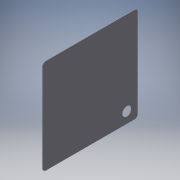
# Autodesk Inventor part: NewFront_C
Saved by Autodesk Inventor 2017 (Build 210142000, 142)
## iProperties
Created: 2019-07-06
Part Number: NewFront_C
Material: Generic
Document SubType Name: Modeling
Designer: DDeGo
Density: 1 g/cm^3
Appearance: Default
Author: DDeGo
Autodesk Inventor part; units mm, degrees
ref_plane "YZ Plane" through (0, 0, 0) normal (1, 0, 0) x (0, 1, 0)
ref_plane "XZ Plane" through (0, 0, 0) normal (0, 1, 0) x (-1, 0, 0)
ref_plane "XY Plane" through (0, 0, 0) normal (0, 0, 1) x (1, 0, 0)
sketch "Sketch1" plane through (0, 0, 0) normal (1, 0, 0) x (0, 1, 0)
  line L0 (0, 13.5) -> (156.5, 13.5) construction
  line L1 (170, 0) -> (170, -156.5) construction
  line L2 (156.5, -170) -> (0, -170) construction
  line L3 (-13.5, -156.5) -> (-13.5, 0) construction
  arc A0 (170, 0) -> (156.5, 13.5) centre (156.5, 0) ccw construction
  arc A1 (156.5, -170) -> (170, -156.5) centre (156.5, -156.5) ccw construction
  arc A2 (-13.5, -156.5) -> (0, -170) centre (0, -156.5) ccw construction
  arc A3 (0, 13.5) -> (-13.5, 0) centre (0, 0) ccw construction
  line L4 (26.5, -21.5) -> (130, -21.5)
  line L5 (135, -26.5) -> (135, -130)
  line L6 (130, -135) -> (26.5, -135)
  line L7 (21.5, -130) -> (21.5, -26.5)
  arc A4 (26.5, -21.5) -> (21.5, -26.5) centre (26.5, -26.5) ccw
  arc A5 (21.5, -130) -> (26.5, -135) centre (26.5, -130) ccw
  arc A6 (130, -135) -> (135, -130) centre (130, -130) ccw
  arc A7 (135, -26.5) -> (130, -21.5) centre (130, -26.5) ccw
  line L8 (156.5, 5.5) -> (0, 5.5)
  arc A8 (0, 5.5) -> (-5.5, 0) centre (0, 0) ccw
  line L9 (-5.5, 0) -> (-5.5, -156.5)
  arc A9 (-5.5, -156.5) -> (0, -162) centre (0, -156.5) ccw
  line L10 (0, -162) -> (156.5, -162)
  arc A10 (156.5, -162) -> (162, -156.5) centre (156.5, -156.5) ccw
  line L11 (162, -156.5) -> (162, 0)
  arc A11 (162, 0) -> (156.5, 5.5) centre (156.5, 0) ccw
  line L12 (17.5, 5.5) -> (17.5, -10.5) construction
  line L13 (14.5, 5.5) -> (14.5, -10.5)
  line L14 (20.5, -10.5) -> (20.5, 5.5)
  arc A12 (20.5, 5.5) -> (14.5, 5.5) centre (17.5, 5.5) ccw
  arc A13 (14.5, -10.5) -> (20.5, -10.5) centre (17.5, -10.5) ccw
  line L15 (31.5455, -10.5) -> (31.5455, 5.5)
  line L16 (28.5455, 5.5) -> (28.5455, -10.5) construction
  arc A14 (25.5455, -10.5) -> (31.5455, -10.5) centre (28.5455, -10.5) ccw
  arc A15 (31.5455, 5.5) -> (25.5455, 5.5) centre (28.5455, 5.5) ccw
  line L17 (25.5455, 5.5) -> (25.5455, -10.5)
  line L18 (42.5909, -10.5) -> (42.5909, 5.5)
  line L19 (39.5909, 5.5) -> (39.5909, -10.5) construction
  arc A16 (36.5909, -10.5) -> (42.5909, -10.5) centre (39.5909, -10.5) ccw
  arc A17 (42.5909, 5.5) -> (36.5909, 5.5) centre (39.5909, 5.5) ccw
  line L20 (36.5909, 5.5) -> (36.5909, -10.5)
  line L21 (53.6364, -10.5) -> (53.6364, 5.5)
  line L22 (50.6364, 5.5) -> (50.6364, -10.5) construction
  arc A18 (47.6364, -10.5) -> (53.6364, -10.5) centre (50.6364, -10.5) ccw
  arc A19 (53.6364, 5.5) -> (47.6364, 5.5) centre (50.6364, 5.5) ccw
  line L23 (47.6364, 5.5) -> (47.6364, -10.5)
  line L24 (64.6818, -10.5) -> (64.6818, 5.5)
  line L25 (61.6818, 5.5) -> (61.6818, -10.5) construction
  arc A20 (58.6818, -10.5) -> (64.6818, -10.5) centre (61.6818, -10.5) ccw
  arc A21 (64.6818, 5.5) -> (58.6818, 5.5) centre (61.6818, 5.5) ccw
  line L26 (58.6818, 5.5) -> (58.6818, -10.5)
  line L27 (75.7273, -10.5) -> (75.7273, 5.5)
  line L28 (72.7273, 5.5) -> (72.7273, -10.5) construction
  arc A22 (69.7273, -10.5) -> (75.7273, -10.5) centre (72.7273, -10.5) ccw
  arc A23 (75.7273, 5.5) -> (69.7273, 5.5) centre (72.7273, 5.5) ccw
  line L29 (69.7273, 5.5) -> (69.7273, -10.5)
  line L30 (86.7727, -10.5) -> (86.7727, 5.5)
  line L31 (83.7727, 5.5) -> (83.7727, -10.5) construction
  arc A24 (80.7727, -10.5) -> (86.7727, -10.5) centre (83.7727, -10.5) ccw
  arc A25 (86.7727, 5.5) -> (80.7727, 5.5) centre (83.7727, 5.5) ccw
  line L32 (80.7727, 5.5) -> (80.7727, -10.5)
  line L33 (97.8182, -10.5) -> (97.8182, 5.5)
  line L34 (94.8182, 5.5) -> (94.8182, -10.5) construction
  arc A26 (91.8182, -10.5) -> (97.8182, -10.5) centre (94.8182, -10.5) ccw
  arc A27 (97.8182, 5.5) -> (91.8182, 5.5) centre (94.8182, 5.5) ccw
  line L35 (91.8182, 5.5) -> (91.8182, -10.5)
  line L36 (108.8636, -10.5) -> (108.8636, 5.5)
  line L37 (105.8636, 5.5) -> (105.8636, -10.5) construction
  arc A28 (102.8636, -10.5) -> (108.8636, -10.5) centre (105.8636, -10.5) ccw
  arc A29 (108.8636, 5.5) -> (102.8636, 5.5) centre (105.8636, 5.5) ccw
  line L38 (102.8636, 5.5) -> (102.8636, -10.5)
  line L39 (119.9091, -10.5) -> (119.9091, 5.5)
  line L40 (116.9091, 5.5) -> (116.9091, -10.5) construction
  arc A30 (113.9091, -10.5) -> (119.9091, -10.5) centre (116.9091, -10.5) ccw
  arc A31 (119.9091, 5.5) -> (113.9091, 5.5) centre (116.9091, 5.5) ccw
  line L41 (113.9091, 5.5) -> (113.9091, -10.5)
  line L42 (130.9545, -10.5) -> (130.9545, 5.5)
  line L43 (127.9545, 5.5) -> (127.9545, -10.5) construction
  arc A32 (124.9545, -10.5) -> (130.9545, -10.5) centre (127.9545, -10.5) ccw
  arc A33 (130.9545, 5.5) -> (124.9545, 5.5) centre (127.9545, 5.5) ccw
  line L44 (124.9545, 5.5) -> (124.9545, -10.5)
  line L45 (142, -10.5) -> (142, 5.5)
  line L46 (139, 5.5) -> (139, -10.5) construction
  arc A34 (136, -10.5) -> (142, -10.5) centre (139, -10.5) ccw
  arc A35 (142, 5.5) -> (136, 5.5) centre (139, 5.5) ccw
  line L47 (136, 5.5) -> (136, -10.5)
  line L48 (26.5, -26.5) -> (130, -130) construction
  arc A36 (10.5, -86.7727) -> (10.5, -80.7727) centre (10.5, -83.7727) ccw
  arc A37 (10.5, -97.8182) -> (10.5, -91.8182) centre (10.5, -94.8182) ccw
  arc A38 (10.5, -119.9091) -> (10.5, -113.9091) centre (10.5, -116.9091) ccw
  arc A39 (10.5, -75.7273) -> (10.5, -69.7273) centre (10.5, -72.7273) ccw
  arc A40 (10.5, -64.6818) -> (10.5, -58.6818) centre (10.5, -61.6818) ccw
  arc A41 (10.5, -53.6364) -> (10.5, -47.6364) centre (10.5, -50.6364) ccw
  arc A42 (10.5, -42.5909) -> (10.5, -36.5909) centre (10.5, -39.5909) ccw
  arc A43 (10.5, -108.8636) -> (10.5, -102.8636) centre (10.5, -105.8636) ccw
  line L49 (10.5, -124.9545) -> (-5.5, -124.9545)
  line L50 (-5.5, -127.9545) -> (10.5, -127.9545) construction
  line L51 (-5.5, -130.9545) -> (10.5, -130.9545)
  arc A44 (-5.5, -124.9545) -> (-5.5, -130.9545) centre (-5.5, -127.9545) ccw
  line L52 (10.5, -136) -> (-5.5, -136)
  line L53 (-5.5, -139) -> (10.5, -139) construction
  arc A45 (-5.5, -136) -> (-5.5, -142) centre (-5.5, -139) ccw
  line L54 (-5.5, -142) -> (10.5, -142)
  arc A46 (10.5, -142) -> (10.5, -136) centre (10.5, -139) ccw
  arc A47 (10.5, -130.9545) -> (10.5, -124.9545) centre (10.5, -127.9545) ccw
  line L55 (-5.5, -119.9091) -> (10.5, -119.9091)
  line L56 (-5.5, -116.9091) -> (10.5, -116.9091) construction
  arc A48 (-5.5, -113.9091) -> (-5.5, -119.9091) centre (-5.5, -116.9091) ccw
  line L57 (10.5, -113.9091) -> (-5.5, -113.9091)
  line L58 (-5.5, -108.8636) -> (10.5, -108.8636)
  line L59 (-5.5, -105.8636) -> (10.5, -105.8636) construction
  line L60 (10.5, -102.8636) -> (-5.5, -102.8636)
  arc A49 (-5.5, -102.8636) -> (-5.5, -108.8636) centre (-5.5, -105.8636) ccw
  line L61 (-5.5, -86.7727) -> (10.5, -86.7727)
  line L62 (-5.5, -83.7727) -> (10.5, -83.7727) construction
  line L63 (10.5, -80.7727) -> (-5.5, -80.7727)
  arc A50 (-5.5, -80.7727) -> (-5.5, -86.7727) centre (-5.5, -83.7727) ccw
  line L64 (-5.5, -75.7273) -> (10.5, -75.7273)
  line L65 (-5.5, -72.7273) -> (10.5, -72.7273) construction
  line L66 (10.5, -69.7273) -> (-5.5, -69.7273)
  arc A51 (-5.5, -69.7273) -> (-5.5, -75.7273) centre (-5.5, -72.7273) ccw
  line L67 (-5.5, -64.6818) -> (10.5, -64.6818)
  line L68 (-5.5, -61.6818) -> (10.5, -61.6818) construction
  line L69 (10.5, -58.6818) -> (-5.5, -58.6818)
  arc A52 (-5.5, -58.6818) -> (-5.5, -64.6818) centre (-5.5, -61.6818) ccw
  line L70 (-5.5, -97.8182) -> (10.5, -97.8182)
  line L71 (-5.5, -94.8182) -> (10.5, -94.8182) construction
  line L72 (10.5, -91.8182) -> (-5.5, -91.8182)
  arc A53 (-5.5, -91.8182) -> (-5.5, -97.8182) centre (-5.5, -94.8182) ccw
  arc A54 (-5.5, -14.5) -> (-5.5, -20.5) centre (-5.5, -17.5) ccw
  line L73 (10.5, -14.5) -> (-5.5, -14.5)
  line L74 (-5.5, -17.5) -> (10.5, -17.5) construction
  line L75 (-5.5, -20.5) -> (10.5, -20.5)
  arc A55 (10.5, -20.5) -> (10.5, -14.5) centre (10.5, -17.5) ccw
  line L76 (-5.5, -28.5455) -> (10.5, -28.5455) construction
  line L77 (-5.5, -31.5455) -> (10.5, -31.5455)
  arc A56 (10.5, -31.5455) -> (10.5, -25.5455) centre (10.5, -28.5455) ccw
  arc A57 (-5.5, -36.5909) -> (-5.5, -42.5909) centre (-5.5, -39.5909) ccw
  line L78 (10.5, -36.5909) -> (-5.5, -36.5909)
  line L79 (-5.5, -39.5909) -> (10.5, -39.5909) construction
  arc A58 (-5.5, -25.5455) -> (-5.5, -31.5455) centre (-5.5, -28.5455) ccw
  line L80 (-5.5, -53.6364) -> (10.5, -53.6364)
  line L81 (-5.5, -50.6364) -> (10.5, -50.6364) construction
  arc A59 (-5.5, -47.6364) -> (-5.5, -53.6364) centre (-5.5, -50.6364) ccw
  line L82 (10.5, -47.6364) -> (-5.5, -47.6364)
  line L83 (-5.5, -42.5909) -> (10.5, -42.5909)
  line L84 (10.5, -25.5455) -> (-5.5, -25.5455)
  arc A60 (86.7727, -146) -> (80.7727, -146) centre (83.7727, -146) ccw
  arc A61 (97.8182, -146) -> (91.8182, -146) centre (94.8182, -146) ccw
  arc A62 (119.9091, -146) -> (113.9091, -146) centre (116.9091, -146) ccw
  arc A63 (75.7273, -146) -> (69.7273, -146) centre (72.7273, -146) ccw
  arc A64 (64.6818, -146) -> (58.6818, -146) centre (61.6818, -146) ccw
  arc A65 (53.6364, -146) -> (47.6364, -146) centre (50.6364, -146) ccw
  arc A66 (42.5909, -146) -> (36.5909, -146) centre (39.5909, -146) ccw
  arc A67 (108.8636, -146) -> (102.8636, -146) centre (105.8636, -146) ccw
  line L85 (124.9545, -146) -> (124.9545, -162)
  line L86 (127.9545, -162) -> (127.9545, -146) construction
  line L87 (130.9545, -162) -> (130.9545, -146)
  arc A68 (124.9545, -162) -> (130.9545, -162) centre (127.9545, -162) ccw
  line L88 (136, -146) -> (136, -162)
  line L89 (139, -162) -> (139, -146) construction
  arc A69 (136, -162) -> (142, -162) centre (139, -162) ccw
  line L90 (142, -162) -> (142, -146)
  arc A70 (142, -146) -> (136, -146) centre (139, -146) ccw
  arc A71 (130.9545, -146) -> (124.9545, -146) centre (127.9545, -146) ccw
  line L91 (119.9091, -162) -> (119.9091, -146)
  line L92 (116.9091, -162) -> (116.9091, -146) construction
  arc A72 (113.9091, -162) -> (119.9091, -162) centre (116.9091, -162) ccw
  line L93 (113.9091, -146) -> (113.9091, -162)
  line L94 (108.8636, -162) -> (108.8636, -146)
  line L95 (105.8636, -162) -> (105.8636, -146) construction
  line L96 (102.8636, -146) -> (102.8636, -162)
  arc A73 (102.8636, -162) -> (108.8636, -162) centre (105.8636, -162) ccw
  line L97 (86.7727, -162) -> (86.7727, -146)
  line L98 (83.7727, -162) -> (83.7727, -146) construction
  line L99 (80.7727, -146) -> (80.7727, -162)
  arc A74 (80.7727, -162) -> (86.7727, -162) centre (83.7727, -162) ccw
  line L100 (75.7273, -162) -> (75.7273, -146)
  line L101 (72.7273, -162) -> (72.7273, -146) construction
  line L102 (69.7273, -146) -> (69.7273, -162)
  arc A75 (69.7273, -162) -> (75.7273, -162) centre (72.7273, -162) ccw
  line L103 (64.6818, -162) -> (64.6818, -146)
  line L104 (61.6818, -162) -> (61.6818, -146) construction
  line L105 (58.6818, -146) -> (58.6818, -162)
  arc A76 (58.6818, -162) -> (64.6818, -162) centre (61.6818, -162) ccw
  line L106 (97.8182, -162) -> (97.8182, -146)
  line L107 (94.8182, -162) -> (94.8182, -146) construction
  line L108 (91.8182, -146) -> (91.8182, -162)
  arc A77 (91.8182, -162) -> (97.8182, -162) centre (94.8182, -162) ccw
  arc A78 (14.5, -162) -> (20.5, -162) centre (17.5, -162) ccw
  line L109 (14.5, -146) -> (14.5, -162)
  line L110 (17.5, -162) -> (17.5, -146) construction
  line L111 (20.5, -162) -> (20.5, -146)
  arc A79 (20.5, -146) -> (14.5, -146) centre (17.5, -146) ccw
  line L112 (28.5455, -162) -> (28.5455, -146) construction
  line L113 (31.5455, -162) -> (31.5455, -146)
  arc A80 (31.5455, -146) -> (25.5455, -146) centre (28.5455, -146) ccw
  arc A81 (36.5909, -162) -> (42.5909, -162) centre (39.5909, -162) ccw
  line L114 (36.5909, -146) -> (36.5909, -162)
  line L115 (39.5909, -162) -> (39.5909, -146) construction
  arc A82 (25.5455, -162) -> (31.5455, -162) centre (28.5455, -162) ccw
  line L116 (53.6364, -162) -> (53.6364, -146)
  line L117 (50.6364, -162) -> (50.6364, -146) construction
  arc A83 (47.6364, -162) -> (53.6364, -162) centre (50.6364, -162) ccw
  line L118 (47.6364, -146) -> (47.6364, -162)
  line L119 (42.5909, -162) -> (42.5909, -146)
  line L120 (25.5455, -146) -> (25.5455, -162)
  arc A84 (146, -69.7273) -> (146, -75.7273) centre (146, -72.7273) ccw
  arc A85 (146, -58.6818) -> (146, -64.6818) centre (146, -61.6818) ccw
  arc A86 (146, -36.5909) -> (146, -42.5909) centre (146, -39.5909) ccw
  arc A87 (146, -80.7727) -> (146, -86.7727) centre (146, -83.7727) ccw
  arc A88 (146, -91.8182) -> (146, -97.8182) centre (146, -94.8182) ccw
  arc A89 (146, -102.8636) -> (146, -108.8636) centre (146, -105.8636) ccw
  arc A90 (146, -113.9091) -> (146, -119.9091) centre (146, -116.9091) ccw
  arc A91 (146, -47.6364) -> (146, -53.6364) centre (146, -50.6364) ccw
  line L121 (146, -31.5455) -> (162, -31.5455)
  line L122 (162, -28.5455) -> (146, -28.5455) construction
  line L123 (162, -25.5455) -> (146, -25.5455)
  arc A92 (162, -31.5455) -> (162, -25.5455) centre (162, -28.5455) ccw
  line L124 (146, -20.5) -> (162, -20.5)
  line L125 (162, -17.5) -> (146, -17.5) construction
  arc A93 (162, -20.5) -> (162, -14.5) centre (162, -17.5) ccw
  line L126 (162, -14.5) -> (146, -14.5)
  arc A94 (146, -14.5) -> (146, -20.5) centre (146, -17.5) ccw
  arc A95 (146, -25.5455) -> (146, -31.5455) centre (146, -28.5455) ccw
  line L127 (162, -36.5909) -> (146, -36.5909)
  line L128 (162, -39.5909) -> (146, -39.5909) construction
  arc A96 (162, -42.5909) -> (162, -36.5909) centre (162, -39.5909) ccw
  line L129 (146, -42.5909) -> (162, -42.5909)
  line L130 (162, -47.6364) -> (146, -47.6364)
  line L131 (162, -50.6364) -> (146, -50.6364) construction
  line L132 (146, -53.6364) -> (162, -53.6364)
  arc A97 (162, -53.6364) -> (162, -47.6364) centre (162, -50.6364) ccw
  line L133 (162, -69.7273) -> (146, -69.7273)
  line L134 (162, -72.7273) -> (146, -72.7273) construction
  line L135 (146, -75.7273) -> (162, -75.7273)
  arc A98 (162, -75.7273) -> (162, -69.7273) centre (162, -72.7273) ccw
  line L136 (162, -80.7727) -> (146, -80.7727)
  line L137 (162, -83.7727) -> (146, -83.7727) construction
  line L138 (146, -86.7727) -> (162, -86.7727)
  arc A99 (162, -86.7727) -> (162, -80.7727) centre (162, -83.7727) ccw
  line L139 (162, -91.8182) -> (146, -91.8182)
  line L140 (162, -94.8182) -> (146, -94.8182) construction
  line L141 (146, -97.8182) -> (162, -97.8182)
  arc A100 (162, -97.8182) -> (162, -91.8182) centre (162, -94.8182) ccw
  line L142 (162, -58.6818) -> (146, -58.6818)
  line L143 (162, -61.6818) -> (146, -61.6818) construction
  line L144 (146, -64.6818) -> (162, -64.6818)
  arc A101 (162, -64.6818) -> (162, -58.6818) centre (162, -61.6818) ccw
  arc A102 (162, -142) -> (162, -136) centre (162, -139) ccw
  line L145 (146, -142) -> (162, -142)
  line L146 (162, -139) -> (146, -139) construction
  line L147 (162, -136) -> (146, -136)
  arc A103 (146, -136) -> (146, -142) centre (146, -139) ccw
  line L148 (162, -127.9545) -> (146, -127.9545) construction
  line L149 (162, -124.9545) -> (146, -124.9545)
  arc A104 (146, -124.9545) -> (146, -130.9545) centre (146, -127.9545) ccw
  arc A105 (162, -119.9091) -> (162, -113.9091) centre (162, -116.9091) ccw
  line L150 (146, -119.9091) -> (162, -119.9091)
  line L151 (162, -116.9091) -> (146, -116.9091) construction
  arc A106 (162, -130.9545) -> (162, -124.9545) centre (162, -127.9545) ccw
  line L152 (162, -102.8636) -> (146, -102.8636)
  line L153 (162, -105.8636) -> (146, -105.8636) construction
  arc A107 (162, -108.8636) -> (162, -102.8636) centre (162, -105.8636) ccw
  line L154 (146, -108.8636) -> (162, -108.8636)
  line L155 (162, -113.9091) -> (146, -113.9091)
  line L156 (146, -130.9545) -> (162, -130.9545)
  point P0 (17.5, -2.5)
  point P1 (28.5455, -2.5)
  point P2 (39.5909, -2.5)
  point P3 (50.6364, -2.5)
  point P4 (61.6818, -2.5)
  point P5 (72.7273, -2.5)
  point P6 (83.7727, -2.5)
  point P7 (94.8182, -2.5)
  point P8 (105.8636, -2.5)
  point P9 (116.9091, -2.5)
  point P10 (127.9545, -2.5)
  point P11 (139, -2.5)
  point P12 (78.25, -78.25)
  point P13 (2.5, -127.9545)
  point P14 (2.5, -139)
  point P15 (2.5, -116.9091)
  point P16 (2.5, -105.8636)
  point P17 (2.5, -83.7727)
  point P18 (2.5, -61.6818)
  point P19 (2.5, -72.7273)
  point P20 (2.5, -94.8182)
  point P21 (2.5, -17.5)
  point P22 (2.5, -28.5455)
  point P23 (2.5, -50.6364)
  point P24 (2.5, -39.5909)
  point P25 (127.9545, -154)
  point P26 (139, -154)
  point P27 (116.9091, -154)
  point P28 (105.8636, -154)
  point P29 (83.7727, -154)
  point P30 (61.6818, -154)
  point P31 (72.7273, -154)
  point P32 (94.8182, -154)
  point P33 (17.5, -154)
  point P34 (28.5455, -154)
  point P35 (50.6364, -154)
  point P36 (39.5909, -154)
  point P37 (154, -28.5455)
  point P38 (154, -17.5)
  point P39 (154, -39.5909)
  point P40 (154, -50.6364)
  point P41 (154, -72.7273)
  point P42 (154, -94.8182)
  point P43 (154, -83.7727)
  point P44 (154, -61.6818)
  point P45 (154, -139)
  point P46 (154, -127.9545)
  point P47 (154, -105.8636)
  point P48 (154, -116.9091)
  dimension "d0" = 13.5
  dimension "d1" = 183.5
  dimension "d2" = 183.5
  dimension "d15" = 35
  dimension "d16" = 35
  dimension "d17" = 35
  dimension "d18" = 35
  dimension "d19" = 5
  dimension "d20" = 8
  dimension "d21" = 16
  dimension "d22" = 3
  dimension "d25" = 11.0455
  dimension "d30" = 20
  dimension "d31" = 20
  dimension "d34" = 360
  dimension "d43" = 167.5
  constraints: 410 end point, 216 point on circle, 108 centre point, 20 tangent, 7 parallel, 6 equal radius, 4 perpendicular, 3 horizontal, 2 midpoint, 1 point on line, 717 other
  measures "d0" radius of A0
  measures "d1" distance between parallel lines of L2 L0
  measures "d2" distance between parallel lines of L1 L3
  measures "d15" distance between parallel lines of L3 L7
  measures "d16" distance between parallel lines of L0 L4
  measures "d17" distance between parallel lines of L1 L5
  measures "d18" distance between parallel lines of L2 L6
  measures "d19" radius of A4
  measures "d20" distance between parallel lines of L0 L8
  measures "d21" distance of L12.start L12.end
  measures "d22" radius of A13
  measures "d25" distance of L14.start L15.start
  measures "d30" distance between parallel lines of L9 L13
  measures "d31" distance between parallel lines of L11 L45
  measures "d43" distance between parallel lines of L9 L11
extrude "Extrusion1" add sketch "Sketch1" along normal blind 1 contours L4 A7 L5 A6 L6 A5 L7 A4 | A11 L11 L126 A94 L124 L123 A95 L121 L127 A86 L129 L130 A91 L132 L142 A85 L144 L133 A84 L135 L136 A87 L138 L139 A88 L141 L152 A89 L154 L155 A90 L150 L149 A104 L156 L147 A103 L145 A10 L10 L90 A70 L88 L87 A71 L85 L91 A62 L93 L94 A67 L96 L106 A61 L108 L97 A60 L99 L100 A63 L102 L103 A64 L105 L116 A65 L118 L119 A66 L114 L113 A80 L120 L111 A79 L109 A9 L9 L54 A46 L52 L51 A47 L49 L55 A38 L57 L58 A43 L60 L70 A37 L72 L61 A36 L63 L64 A39 L66 L67 A40 L69 L80 A41 L82 L83 A42 L78 L77 A56 L84 L75 A55 L73 A8 L8 L13 A13 L14 L17 A14 L15 L20 A16 L18 L23 A18 L21 L26 A20 L24 L29 A22 L27 L32 A24 L30 L35 A26 L33 L38 A28 L36 L41 A30 L39 L44 A32 L42 L47 A34 L45 | L45 A34 L47 L8 | L11 L124 A94 L126 | L42 A32 L44 L8 | L11 L121 A95 L123 | L39 A30 L41 L8 | L11 L129 A86 L127 | L36 A28 L38 L8 | L11 L132 A91 L130 | L33 A26 L35 L8 | L11 L144 A85 L142 | L30 A24 L32 L8 | L11 L135 A84 L133 | L27 A22 L29 L8 | L11 L138 A87 L136 | L24 A20 L26 L8 | L11 L141 A88 L139 | L21 A18 L23 L8 | L11 L154 A89 L152 | L18 A16 L20 L8 | L11 L150 A90 L155 | L15 A14 L17 L8 | L11 L156 A104 L149 | L14 A13 L13 L8 | L11 L145 A103 L147 | L73 A55 L75 L9 | L10 L88 A70 L90 | L84 A56 L77 L9 | L10 L85 A71 L87 | L78 A42 L83 L9 | L10 L93 A62 L91 | L82 A41 L80 L9 | L10 L96 A67 L94 | L69 A40 L67 L9 | L10 L108 A61 L106 | L66 A39 L64 L9 | L10 L99 A60 L97 | L63 A36 L61 L9 | L10 L102 A63 L100 | L72 A37 L70 L9 | L10 L105 A64 L103 | L60 A43 L58 L9 | L10 L118 A65 L116 | L57 A38 L55 L9 | L10 L114 A66 L119 | L49 A47 L51 L9 | L10 L120 A80 L113 | L52 A46 L54 L9 | L10 L109 A79 L111
sketch "Sketch2" plane through (1, 0, 0) normal (1, 0, 0) x (0, 0, -1)
  circle A0 centre (143, 143) radius 8.1
  line L0 (156.5, 162) -> (0, 162) projected
  line L1 (162, 0) -> (162, 156.5) projected
  point P0 (0, 0)
  dimension "d38" = 19
  dimension "d39" = 19
  dimension "d40" = 16.2
  constraints: 1 centre point
  measures "d38" distance from line of L0 A0.centre
  measures "d39" distance from line of L1 A0.centre
  measures "d40" diameter of A0
extrude "Extrusion3" cut sketch "Sketch2" against normal blind 10
equation "\"d2\" = d1"
equation "\"d16\" = d15"
equation "\"d17\" = d15"
equation "\"d18\" = d15"
body "Solid1"
